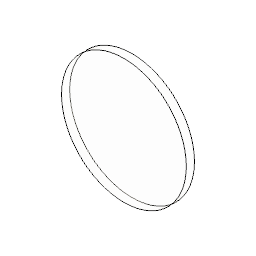
Lens D-Cx Dia38mm FL50mm (Autodesk Fusion 360 design; units mm, degrees)
Autodesk Fusion 360 part; units mm, degrees
sketch "Sketch1" plane through (0, 0, 0) normal (1, 0, 0) x (0, 1, 0)
  line L0 (-5, 5) -> (5, 5) construction
  line L1 (0, 5) -> (0, 24) construction
  line L2 (0, 24) -> (1.2493, 24) construction
  line L3 (1.2493, 24) -> (-1.2493, 24) construction
  line L4 (-1.2493, 24) -> (1.2493, 24) construction
  line L5 (-1.2493, 24) -> (1.2493, 24)
  arc A0 (-1.2493, 24) -> (-5, 5) centre (45, 5) ccw
  arc A1 (5, 5) -> (1.2493, 24) centre (-45, 5) ccw
  line L6 (-5, 5) -> (5, 5)
  constraint midpoint L0 L1.start
  constraint perpendicular L0 L1
  constraint perpendicular L1 L2
  constraint perpendicular L1 L3
revolve "Revolve1" add sketch "Sketch1" angle 360 about axis through (0, -5, 5) along (0, 1, 0)
move_body "Move1" bodies 1 to x (1, 0, 0) y (0, 1, 0) z (0, 0, 1) at (0, 0, 13)
move_body "Move2" bodies 1 to x (1, 0, 0) y (0, 1, 0) z (0, 0, 1) at (0, 0, 10)
move_body "Move3" bodies 1 to x (1, 0, 0) y (0, 1, 0) z (0, 0, 1) at (0, 0, -9)
move_body "Move4" bodies 1 to x (1, 0, 0) y (0, 1, 0) z (0, 0, 1) at (0, 0, -19)
